Autodesk Fusion 360 part; units mm, degrees
(part 2 of 3)
  arc A16 (-17.9906, -30.6144) -> (-8.9264, -34.3689) centre (0, 0) ccw
  arc A17 (-7.7732, -36.2381) -> (-8.9264, -34.3689) centre (-9.3255, -35.9054) ccw
  line L8 (-7.7732, -36.2381) -> (-10.0097, -46.6751)
  spline S8 degree 5 poles (-10.0097, -46.6751) (-10.0198, -46.7226) (-10.0383, -46.8178) (-10.0605, -46.9612) (-10.0796, -47.1537) (-10.0893, -47.3962) (-10.0891, -47.6398) (-10.0829, -47.8842) (-10.0736, -48.129) (-10.0619, -48.374) (-10.0476, -48.6191) (-10.0296, -48.8645) (-10.007, -49.1102) (-9.9792, -49.3562) (-9.9463, -49.6025) (-9.9089, -49.849) (-9.8676, -50.0955) (-9.8231, -50.3422) (-9.7758, -50.5887) (-9.7255, -50.8353) (-9.6724, -51.0817) (-9.6161, -51.3281) (-9.5567, -51.5744) (-9.4939, -51.8206) (-9.428, -52.0667) (-9.3591, -52.3127) (-9.2873, -52.5584) (-9.2128, -52.804) (-9.1355, -53.0494) (-9.0557, -53.2944) (-8.9732, -53.5393) (-8.8881, -53.7839) (-8.8003, -54.0281) (-8.71, -54.2721) (-8.617, -54.5158) (-8.5215, -54.7591) (-8.4236, -55.0021) (-8.3232, -55.2447) (-8.2204, -55.487) (-8.1152, -55.7288) (-8.0077, -55.9702) (-7.8978, -56.2112) (-7.7856, -56.4518) (-7.6711, -56.6919) (-7.5543, -56.9315) (-7.4353, -57.1707) (-7.314, -57.4094) (-7.1905, -57.6476) (-7.0648, -57.8853) (-6.937, -58.1224) (-6.807, -58.3591) (-6.6749, -58.5951) (-6.5406, -58.8307) (-6.4043, -59.0656) (-6.2659, -59.3) (-6.1254, -59.5337) (-5.9828, -59.7669) (-5.8383, -59.9994) (-5.6917, -60.2314) (-5.5431, -60.4627) (-5.3925, -60.6933) (-5.24, -60.9233) (-5.0855, -61.1526) (-4.929, -61.3813) (-4.7706, -61.6093) (-4.6103, -61.8365) (-4.4481, -62.0631) (-4.2841, -62.2889) (-4.1181, -62.5141) (-3.9503, -62.7384) (-3.7806, -62.9621) (-3.6434, -63.1404) (-3.5397, -63.2738) (-3.4702, -63.3626) (-3.4353, -63.407) knots 0 0 0 0 0 0 0.01428571 0.02857143 0.04285714 0.05714286 0.07142857 0.08571429 0.1 0.11428571 0.12857143 0.14285714 0.15714286 0.17142857 0.18571429 0.2 0.21428571 0.22857143 0.24285714 0.25714286 0.27142857 0.28571429 0.3 0.31428571 0.32857143 0.34285714 0.35714286 0.37142857 0.38571429 0.4 0.41428571 0.42857143 0.44285714 0.45714286 0.47142857 0.48571429 0.5 0.51428571 0.52857143 0.54285714 0.55714286 0.57142857 0.58571429 0.6 0.61428571 0.62857143 0.64285714 0.65714286 0.67142857 0.68571429 0.7 0.71428571 0.72857143 0.74285714 0.75714286 0.77142857 0.78571429 0.8 0.81428571 0.82857143 0.84285714 0.85714286 0.87142857 0.88571429 0.9 0.91428571 0.92857143 0.94285714 0.95714286 0.97142857 0.98571429 1 1 1 1 1 1
  arc A18 (-3.4353, -63.407) -> (3.4353, -63.407) centre (0, 0) ccw
  spline S9 degree 5 poles (10.0097, -46.6751) (10.0198, -46.7226) (10.0383, -46.8178) (10.0605, -46.9612) (10.0796, -47.1537) (10.0893, -47.3962) (10.0891, -47.6398) (10.0829, -47.8842) (10.0736, -48.129) (10.0619, -48.374) (10.0476, -48.6191) (10.0296, -48.8645) (10.007, -49.1102) (9.9792, -49.3562) (9.9463, -49.6025) (9.9089, -49.849) (9.8676, -50.0955) (9.8231, -50.3422) (9.7758, -50.5887) (9.7255, -50.8353) (9.6724, -51.0817) (9.6161, -51.3281) (9.5567, -51.5744) (9.4939, -51.8206) (9.428, -52.0667) (9.3591, -52.3127) (9.2873, -52.5584) (9.2128, -52.804) (9.1355, -53.0494) (9.0557, -53.2944) (8.9732, -53.5393) (8.8881, -53.7839) (8.8003, -54.0281) (8.71, -54.2721) (8.617, -54.5158) (8.5215, -54.7591) (8.4236, -55.0021) (8.3232, -55.2447) (8.2204, -55.487) (8.1152, -55.7288) (8.0077, -55.9702) (7.8978, -56.2112) (7.7856, -56.4518) (7.6711, -56.6919) (7.5543, -56.9315) (7.4353, -57.1707) (7.314, -57.4094) (7.1905, -57.6476) (7.0648, -57.8853) (6.937, -58.1224) (6.807, -58.3591) (6.6749, -58.5951) (6.5406, -58.8307) (6.4043, -59.0656) (6.2659, -59.3) (6.1254, -59.5337) (5.9828, -59.7669) (5.8383, -59.9994) (5.6917, -60.2314) (5.5431, -60.4627) (5.3925, -60.6933) (5.24, -60.9233) (5.0855, -61.1526) (4.929, -61.3813) (4.7706, -61.6093) (4.6103, -61.8365) (4.4481, -62.0631) (4.2841, -62.2889) (4.1181, -62.5141) (3.9503, -62.7384) (3.7806, -62.9621) (3.6434, -63.1404) (3.5397, -63.2738) (3.4702, -63.3626) (3.4353, -63.407) knots 0 0 0 0 0 0 0.01428571 0.02857143 0.04285714 0.05714286 0.07142857 0.08571429 0.1 0.11428571 0.12857143 0.14285714 0.15714286 0.17142857 0.18571429 0.2 0.21428571 0.22857143 0.24285714 0.25714286 0.27142857 0.28571429 0.3 0.31428571 0.32857143 0.34285714 0.35714286 0.37142857 0.38571429 0.4 0.41428571 0.42857143 0.44285714 0.45714286 0.47142857 0.48571429 0.5 0.51428571 0.52857143 0.54285714 0.55714286 0.57142857 0.58571429 0.6 0.61428571 0.62857143 0.64285714 0.65714286 0.67142857 0.68571429 0.7 0.71428571 0.72857143 0.74285714 0.75714286 0.77142857 0.78571429 0.8 0.81428571 0.82857143 0.84285714 0.85714286 0.87142857 0.88571429 0.9 0.91428571 0.92857143 0.94285714 0.95714286 0.97142857 0.98571429 1 1 1 1 1 1
  line L9 (10.0097, -46.6751) -> (7.7732, -36.2381)
  arc A19 (8.9264, -34.3689) -> (7.7732, -36.2381) centre (9.3255, -35.9054) ccw
  arc A20 (8.9264, -34.3689) -> (17.9906, -30.6144) centre (0, 0) ccw
  arc A21 (20.1277, -31.1207) -> (17.9906, -30.6144) centre (18.7949, -31.9831) ccw
  line L10 (20.1277, -31.1207) -> (25.9264, -40.0822)
  spline S10 degree 5 poles (25.9264, -40.0822) (25.9528, -40.123) (26.007, -40.2033) (26.0927, -40.3204) (26.2154, -40.4701) (26.3799, -40.6484) (26.5524, -40.8205) (26.7296, -40.989) (26.9092, -41.1554) (27.0907, -41.3204) (27.2742, -41.4836) (27.4604, -41.6444) (27.6501, -41.8022) (27.8437, -41.9565) (28.0411, -42.1074) (28.2419, -42.2552) (28.4454, -42.4004) (28.6513, -42.5433) (28.8591, -42.6841) (29.069, -42.823) (29.2808, -42.9596) (29.4948, -43.0941) (29.711, -43.2262) (29.9295, -43.3559) (30.1501, -43.4833) (30.3728, -43.6085) (30.5973, -43.7315) (30.8237, -43.8525) (31.0517, -43.9714) (31.2815, -44.0882) (31.513, -44.203) (31.7461, -44.3158) (31.9809, -44.4264) (32.2173, -44.5351) (32.4553, -44.6416) (32.6949, -44.7462) (32.936, -44.8487) (33.1785, -44.9493) (33.4225, -45.0479) (33.6679, -45.1445) (33.9146, -45.2392) (34.1627, -45.3319) (34.4122, -45.4227) (34.6629, -45.5115) (34.915, -45.5984) (35.1683, -45.6833) (35.4228, -45.7664) (35.6786, -45.8475) (35.9355, -45.9267) (36.1936, -46.004) (36.4528, -46.0794) (36.7132, -46.1529) (36.9746, -46.2245) (37.2372, -46.2942) (37.5008, -46.362) (37.7654, -46.428) (38.0311, -46.4921) (38.2977, -46.5543) (38.5654, -46.6146) (38.834, -46.6731) (39.1036, -46.7297) (39.3741, -46.7845) (39.6455, -46.8374) (39.9178, -46.8885) (40.191, -46.9377) (40.465, -46.985) (40.7399, -47.0305) (41.0156, -47.0742) (41.2922, -47.1161) (41.5695, -47.1561) (41.8476, -47.1942) (42.0707, -47.2233) (42.2384, -47.2443) (42.3504, -47.2579) (42.4064, -47.2647) knots 0 0 0 0 0 0 0.01428571 0.02857143 0.04285714 0.05714286 0.07142857 0.08571429 0.1 0.11428571 0.12857143 0.14285714 0.15714286 0.17142857 0.18571429 0.2 0.21428571 0.22857143 0.24285714 0.25714286 0.27142857 0.28571429 0.3 0.31428571 0.32857143 0.34285714 0.35714286 0.37142857 0.38571429 0.4 0.41428571 0.42857143 0.44285714 0.45714286 0.47142857 0.48571429 0.5 0.51428571 0.52857143 0.54285714 0.55714286 0.57142857 0.58571429 0.6 0.61428571 0.62857143 0.64285714 0.65714286 0.67142857 0.68571429 0.7 0.71428571 0.72857143 0.74285714 0.75714286 0.77142857 0.78571429 0.8 0.81428571 0.82857143 0.84285714 0.85714286 0.87142857 0.88571429 0.9 0.91428571 0.92857143 0.94285714 0.95714286 0.97142857 0.98571429 1 1 1 1 1 1
  arc A22 (42.4064, -47.2647) -> (47.2647, -42.4064) centre (0, 0) ccw
  spline S11 degree 5 poles (40.0822, -25.9264) (40.123, -25.9528) (40.2033, -26.007) (40.3204, -26.0927) (40.4701, -26.2154) (40.6484, -26.3799) (40.8205, -26.5524) (40.989, -26.7296) (41.1554, -26.9092) (41.3204, -27.0907) (41.4836, -27.2742) (41.6444, -27.4604) (41.8022, -27.6501) (41.9565, -27.8437) (42.1074, -28.0411) (42.2552, -28.2419) (42.4004, -28.4454) (42.5433, -28.6513) (42.6841, -28.8591) (42.823, -29.069) (42.9596, -29.2808) (43.0941, -29.4948) (43.2262, -29.711) (43.3559, -29.9295) (43.4833, -30.1501) (43.6085, -30.3728) (43.7315, -30.5973) (43.8525, -30.8237) (43.9714, -31.0517) (44.0882, -31.2815) (44.203, -31.513) (44.3158, -31.7461) (44.4264, -31.9809) (44.5351, -32.2173) (44.6416, -32.4553) (44.7462, -32.6949) (44.8487, -32.936) (44.9493, -33.1785) (45.0479, -33.4225) (45.1445, -33.6679) (45.2392, -33.9146) (45.3319, -34.1627) (45.4227, -34.4122) (45.5115, -34.6629) (45.5984, -34.915) (45.6833, -35.1683) (45.7664, -35.4228) (45.8475, -35.6786) (45.9267, -35.9355) (46.004, -36.1936) (46.0794, -36.4528) (46.1529, -36.7132) (46.2245, -36.9746) (46.2942, -37.2372) (46.362, -37.5008) (46.428, -37.7654) (46.4921, -38.0311) (46.5543, -38.2977) (46.6146, -38.5654) (46.6731, -38.834) (46.7297, -39.1036) (46.7845, -39.3741) (46.8374, -39.6455) (46.8885, -39.9178) (46.9377, -40.191) (46.985, -40.465) (47.0305, -40.7399) (47.0742, -41.0156) (47.1161, -41.2922) (47.1561, -41.5695) (47.1942, -41.8476) (47.2233, -42.0707) (47.2443, -42.2384) (47.2579, -42.3504) (47.2647, -42.4064) knots 0 0 0 0 0 0 0.01428571 0.02857143 0.04285714 0.05714286 0.07142857 0.08571429 0.1 0.11428571 0.12857143 0.14285714 0.15714286 0.17142857 0.18571429 0.2 0.21428571 0.22857143 0.24285714 0.25714286 0.27142857 0.28571429 0.3 0.31428571 0.32857143 0.34285714 0.35714286 0.37142857 0.38571429 0.4 0.41428571 0.42857143 0.44285714 0.45714286 0.47142857 0.48571429 0.5 0.51428571 0.52857143 0.54285714 0.55714286 0.57142857 0.58571429 0.6 0.61428571 0.62857143 0.64285714 0.65714286 0.67142857 0.68571429 0.7 0.71428571 0.72857143 0.74285714 0.75714286 0.77142857 0.78571429 0.8 0.81428571 0.82857143 0.84285714 0.85714286 0.87142857 0.88571429 0.9 0.91428571 0.92857143 0.94285714 0.95714286 0.97142857 0.98571429 1 1 1 1 1 1
  line L11 (40.0822, -25.9264) -> (31.1207, -20.1277)
  arc A23 (30.6144, -17.9906) -> (31.1207, -20.1277) centre (31.9831, -18.7949) ccw
  arc A24 (30.6144, -17.9906) -> (34.3689, -8.9264) centre (0, 0) ccw
  arc A25 (36.2381, -7.7732) -> (34.3689, -8.9264) centre (35.9054, -9.3255) ccw
  line L12 (36.2381, -7.7732) -> (46.6751, -10.0097)
  spline S12 degree 5 poles (46.6751, -10.0097) (46.7226, -10.0198) (46.8178, -10.0383) (46.9612, -10.0605) (47.1537, -10.0796) (47.3962, -10.0893) (47.6398, -10.0891) (47.8842, -10.0829) (48.129, -10.0736) (48.374, -10.0619) (48.6191, -10.0476) (48.8645, -10.0296) (49.1102, -10.007) (49.3562, -9.9792) (49.6025, -9.9463) (49.849, -9.9089) (50.0955, -9.8676) (50.3422, -9.8231) (50.5887, -9.7758) (50.8353, -9.7255) (51.0817, -9.6724) (51.3281, -9.6161) (51.5744, -9.5567) (51.8206, -9.4939) (52.0667, -9.428) (52.3127, -9.3591) (52.5584, -9.2873) (52.804, -9.2128) (53.0494, -9.1355) (53.2944, -9.0557) (53.5393, -8.9732) (53.7839, -8.8881) (54.0281, -8.8003) (54.2721, -8.71) (54.5158, -8.617) (54.7591, -8.5215) (55.0021, -8.4236) (55.2447, -8.3232) (55.487, -8.2204) (55.7288, -8.1152) (55.9702, -8.0077) (56.2112, -7.8978) (56.4518, -7.7856) (56.6919, -7.6711) (56.9315, -7.5543) (57.1707, -7.4353) (57.4094, -7.314) (57.6476, -7.1905) (57.8853, -7.0648) (58.1224, -6.937) (58.3591, -6.807) (58.5951, -6.6749) (58.8307, -6.5406) (59.0656, -6.4043) (59.3, -6.2659) (59.5337, -6.1254) (59.7669, -5.9828) (59.9994, -5.8383) (60.2314, -5.6917) (60.4627, -5.5431) (60.6933, -5.3925) (60.9233, -5.24) (61.1526, -5.0855) (61.3813, -4.929) (61.6093, -4.7706) (61.8365, -4.6103) (62.0631, -4.4481) (62.2889, -4.2841) (62.5141, -4.1181) (62.7384, -3.9503) (62.9621, -3.7806) (63.1404, -3.6434) (63.2738, -3.5397) (63.3626, -3.4702) (63.407, -3.4353) knots 0 0 0 0 0 0 0.01428571 0.02857143 0.04285714 0.05714286 0.07142857 0.08571429 0.1 0.11428571 0.12857143 0.14285714 0.15714286 0.17142857 0.18571429 0.2 0.21428571 0.22857143 0.24285714 0.25714286 0.27142857 0.28571429 0.3 0.31428571 0.32857143 0.34285714 0.35714286 0.37142857 0.38571429 0.4 0.41428571 0.42857143 0.44285714 0.45714286 0.47142857 0.48571429 0.5 0.51428571 0.52857143 0.54285714 0.55714286 0.57142857 0.58571429 0.6 0.61428571 0.62857143 0.64285714 0.65714286 0.67142857 0.68571429 0.7 0.71428571 0.72857143 0.74285714 0.75714286 0.77142857 0.78571429 0.8 0.81428571 0.82857143 0.84285714 0.85714286 0.87142857 0.88571429 0.9 0.91428571 0.92857143 0.94285714 0.95714286 0.97142857 0.98571429 1 1 1 1 1 1
  arc A26 (63.407, -3.4353) -> (63.407, 3.4353) centre (0, 0) ccw
  spline S13 degree 5 poles (46.6751, 10.0097) (46.7226, 10.0198) (46.8178, 10.0383) (46.9612, 10.0605) (47.1537, 10.0796) (47.3962, 10.0893) (47.6398, 10.0891) (47.8842, 10.0829) (48.129, 10.0736) (48.374, 10.0619) (48.6191, 10.0476) (48.8645, 10.0296) (49.1102, 10.007) (49.3562, 9.9792) (49.6025, 9.9463) (49.849, 9.9089) (50.0955, 9.8676) (50.3422, 9.8231) (50.5887, 9.7758) (50.8353, 9.7255) (51.0817, 9.6724) (51.3281, 9.6161) (51.5744, 9.5567) (51.8206, 9.4939) (52.0667, 9.428) (52.3127, 9.3591) (52.5584, 9.2873) (52.804, 9.2128) (53.0494, 9.1355) (53.2944, 9.0557) (53.5393, 8.9732) (53.7839, 8.8881) (54.0281, 8.8003) (54.2721, 8.71) (54.5158, 8.617) (54.7591, 8.5215) (55.0021, 8.4236) (55.2447, 8.3232) (55.487, 8.2204) (55.7288, 8.1152) (55.9702, 8.0077) (56.2112, 7.8978) (56.4518, 7.7856) (56.6919, 7.6711) (56.9315, 7.5543) (57.1707, 7.4353) (57.4094, 7.314) (57.6476, 7.1905) (57.8853, 7.0648) (58.1224, 6.937) (58.3591, 6.807) (58.5951, 6.6749) (58.8307, 6.5406) (59.0656, 6.4043) (59.3, 6.2659) (59.5337, 6.1254) (59.7669, 5.9828) (59.9994, 5.8383) (60.2314, 5.6917) (60.4627, 5.5431) (60.6933, 5.3925) (60.9233, 5.24) (61.1526, 5.0855) (61.3813, 4.929) (61.6093, 4.7706) (61.8365, 4.6103) (62.0631, 4.4481) (62.2889, 4.2841) (62.5141, 4.1181) (62.7384, 3.9503) (62.9621, 3.7806) (63.1404, 3.6434) (63.2738, 3.5397) (63.3626, 3.4702) (63.407, 3.4353) knots 0 0 0 0 0 0 0.01428571 0.02857143 0.04285714 0.05714286 0.07142857 0.08571429 0.1 0.11428571 0.12857143 0.14285714 0.15714286 0.17142857 0.18571429 0.2 0.21428571 0.22857143 0.24285714 0.25714286 0.27142857 0.28571429 0.3 0.31428571 0.32857143 0.34285714 0.35714286 0.37142857 0.38571429 0.4 0.41428571 0.42857143 0.44285714 0.45714286 0.47142857 0.48571429 0.5 0.51428571 0.52857143 0.54285714 0.55714286 0.57142857 0.58571429 0.6 0.61428571 0.62857143 0.64285714 0.65714286 0.67142857 0.68571429 0.7 0.71428571 0.72857143 0.74285714 0.75714286 0.77142857 0.78571429 0.8 0.81428571 0.82857143 0.84285714 0.85714286 0.87142857 0.88571429 0.9 0.91428571 0.92857143 0.94285714 0.95714286 0.97142857 0.98571429 1 1 1 1 1 1
  line L13 (46.6751, 10.0097) -> (36.2381, 7.7732)
  arc A27 (34.3689, 8.9264) -> (36.2381, 7.7732) centre (35.9054, 9.3255) ccw
  arc A28 (34.3689, 8.9264) -> (30.6144, 17.9906) centre (0, 0) ccw
  arc A29 (31.1207, 20.1277) -> (30.6144, 17.9906) centre (31.9831, 18.7949) ccw
  line L14 (31.1207, 20.1277) -> (40.0822, 25.9264)
  spline S14 degree 5 poles (40.0822, 25.9264) (40.123, 25.9528) (40.2033, 26.007) (40.3204, 26.0927) (40.4701, 26.2154) (40.6484, 26.3799) (40.8205, 26.5524) (40.989, 26.7296) (41.1554, 26.9092) (41.3204, 27.0907) (41.4836, 27.2742) (41.6444, 27.4604) (41.8022, 27.6501) (41.9565, 27.8437) (42.1074, 28.0411) (42.2552, 28.2419) (42.4004, 28.4454) (42.5433, 28.6513) (42.6841, 28.8591) (42.823, 29.069) (42.9596, 29.2808) (43.0941, 29.4948) (43.2262, 29.711) (43.3559, 29.9295) (43.4833, 30.1501) (43.6085, 30.3728) (43.7315, 30.5973) (43.8525, 30.8237) (43.9714, 31.0517) (44.0882, 31.2815) (44.203, 31.513) (44.3158, 31.7461) (44.4264, 31.9809) (44.5351, 32.2173) (44.6416, 32.4553) (44.7462, 32.6949) (44.8487, 32.936) (44.9493, 33.1785) (45.0479, 33.4225) (45.1445, 33.6679) (45.2392, 33.9146) (45.3319, 34.1627) (45.4227, 34.4122) (45.5115, 34.6629) (45.5984, 34.915) (45.6833, 35.1683) (45.7664, 35.4228) (45.8475, 35.6786) (45.9267, 35.9355) (46.004, 36.1936) (46.0794, 36.4528) (46.1529, 36.7132) (46.2245, 36.9746) (46.2942, 37.2372) (46.362, 37.5008) (46.428, 37.7654) (46.4921, 38.0311) (46.5543, 38.2977) (46.6146, 38.5654) (46.6731, 38.834) (46.7297, 39.1036) (46.7845, 39.3741) (46.8374, 39.6455) (46.8885, 39.9178) (46.9377, 40.191) (46.985, 40.465) (47.0305, 40.7399) (47.0742, 41.0156) (47.1161, 41.2922) (47.1561, 41.5695) (47.1942, 41.8476) (47.2233, 42.0707) (47.2443, 42.2384) (47.2579, 42.3504) (47.2647, 42.4064) knots 0 0 0 0 0 0 0.01428571 0.02857143 0.04285714 0.05714286 0.07142857 0.08571429 0.1 0.11428571 0.12857143 0.14285714 0.15714286 0.17142857 0.18571429 0.2 0.21428571 0.22857143 0.24285714 0.25714286 0.27142857 0.28571429 0.3 0.31428571 0.32857143 0.34285714 0.35714286 0.37142857 0.38571429 0.4 0.41428571 0.42857143 0.44285714 0.45714286 0.47142857 0.48571429 0.5 0.51428571 0.52857143 0.54285714 0.55714286 0.57142857 0.58571429 0.6 0.61428571 0.62857143 0.64285714 0.65714286 0.67142857 0.68571429 0.7 0.71428571 0.72857143 0.74285714 0.75714286 0.77142857 0.78571429 0.8 0.81428571 0.82857143 0.84285714 0.85714286 0.87142857 0.88571429 0.9 0.91428571 0.92857143 0.94285714 0.95714286 0.97142857 0.98571429 1 1 1 1 1 1
  arc A30 (47.2647, 42.4064) -> (42.4064, 47.2647) centre (0, 0) ccw
  spline S15 degree 5 poles (25.9264, 40.0822) (25.9528, 40.123) (26.007, 40.2033) (26.0927, 40.3204) (26.2154, 40.4701) (26.3799, 40.6484) (26.5524, 40.8205) (26.7296, 40.989) (26.9092, 41.1554) (27.0907, 41.3204) (27.2742, 41.4836) (27.4604, 41.6444) (27.6501, 41.8022) (27.8437, 41.9565) (28.0411, 42.1074) (28.2419, 42.2552) (28.4454, 42.4004) (28.6513, 42.5433) (28.8591, 42.6841) (29.069, 42.823) (29.2808, 42.9596) (29.4948, 43.0941) (29.711, 43.2262) (29.9295, 43.3559) (30.1501, 43.4833) (30.3728, 43.6085) (30.5973, 43.7315) (30.8237, 43.8525) (31.0517, 43.9714) (31.2815, 44.0882) (31.513, 44.203) (31.7461, 44.3158) (31.9809, 44.4264) (32.2173, 44.5351) (32.4553, 44.6416) (32.6949, 44.7462) (32.936, 44.8487) (33.1785, 44.9493) (33.4225, 45.0479) (33.6679, 45.1445) (33.9146, 45.2392) (34.1627, 45.3319) (34.4122, 45.4227) (34.6629, 45.5115) (34.915, 45.5984) (35.1683, 45.6833) (35.4228, 45.7664) (35.6786, 45.8475) (35.9355, 45.9267) (36.1936, 46.004) (36.4528, 46.0794) (36.7132, 46.1529) (36.9746, 46.2245) (37.2372, 46.2942) (37.5008, 46.362) (37.7654, 46.428) (38.0311, 46.4921) (38.2977, 46.5543) (38.5654, 46.6146) (38.834, 46.6731) (39.1036, 46.7297) (39.3741, 46.7845) (39.6455, 46.8374) (39.9178, 46.8885) (40.191, 46.9377) (40.465, 46.985) (40.7399, 47.0305) (41.0156, 47.0742) (41.2922, 47.1161) (41.5695, 47.1561) (41.8476, 47.1942) (42.0707, 47.2233) (42.2384, 47.2443) (42.3504, 47.2579) (42.4064, 47.2647) knots 0 0 0 0 0 0 0.01428571 0.02857143 0.04285714 0.05714286 0.07142857 0.08571429 0.1 0.11428571 0.12857143 0.14285714 0.15714286 0.17142857 0.18571429 0.2 0.21428571 0.22857143 0.24285714 0.25714286 0.27142857 0.28571429 0.3 0.31428571 0.32857143 0.34285714 0.35714286 0.37142857 0.38571429 0.4 0.41428571 0.42857143 0.44285714 0.45714286 0.47142857 0.48571429 0.5 0.51428571 0.52857143 0.54285714 0.55714286 0.57142857 0.58571429 0.6 0.61428571 0.62857143 0.64285714 0.65714286 0.67142857 0.68571429 0.7 0.71428571 0.72857143 0.74285714 0.75714286 0.77142857 0.78571429 0.8 0.81428571 0.82857143 0.84285714 0.85714286 0.87142857 0.88571429 0.9 0.91428571 0.92857143 0.94285714 0.95714286 0.97142857 0.98571429 1 1 1 1 1 1
  line L15 (25.9264, 40.0822) -> (20.1277, 31.1207)
  arc A31 (17.9906, 30.6144) -> (20.1277, 31.1207) centre (18.7949, 31.9831) ccw
  arc A32 (17.9906, 30.6144) -> (8.9264, 34.3689) centre (0, 0) ccw
  circle A33 centre (0, 0) radius 7
  circle A34 centre (0, 0) radius 10
  line L16 (0, 13) -> (0, -12)
  circle A35 centre (0, 0) radius 27.5
  circle A36 centre (0, 0) radius 15
  line L17 (0, 0) -> (-5.1303, 14.0954)
  line L18 (0, 0) -> (5.1303, 14.0954)
  line L19 (-5.1303, 14.0954) -> (-9.4056, 25.8415)
  line L20 (5.1303, 14.0954) -> (9.4056, 25.8415)
  line L21 (-14.7721, 2.6047) -> (-27.0822, 4.7753)
  line L22 (-9.6418, 11.4907) -> (-17.6767, 21.0662)
  line L23 (-9.6418, -11.4907) -> (-17.6767, -21.0662)
  line L24 (-14.7721, -2.6047) -> (-27.0822, -4.7753)
  line L25 (5.1303, -14.0954) -> (9.4056, -25.8415)
  line L26 (-5.1303, -14.0954) -> (-9.4056, -25.8415)
  line L27 (14.7721, -2.6047) -> (27.0822, -4.7753)
  line L28 (9.6418, -11.4907) -> (17.6767, -21.0662)
  line L29 (9.6418, 11.4907) -> (17.6767, 21.0662)
  line L30 (14.7721, 2.6047) -> (27.0822, 4.7753)
  point P0 (0, 7)
  dimension "d25" = 14
  dimension "d30" = 3
  dimension "d37" = 55
  dimension "d38" = 30
  dimension "d39" = 40
  dimension "d40" = 20
  dimension "d42" = 360
  constraint concentric A0 A33
  constraint vertical L16
  constraint coincident A0.centre L16
  constraint coincident L16 P0
  constraint coincident A33 P0
  constraint concentric A33 A35
  constraint concentric A33 A36
  constraint coincident A0.centre A2.centre
  constraint coincident A35 L19.end
  constraint coincident A35 L20.end
  constraint coincident A36 L17.end
  constraint coincident A36 L18.end
  measures "d25" diameter of A33
  measures "d37" diameter of A35
  measures "d38" diameter of A36
  measures "d39" angle of L17 L18
  measures "d40" angle of L16 L18
extrude "Extrude3" cut sketch "Sketch1 (3)" against normal up to surface (32.7 mm away) contours A0 A33 L16 L18 | A0 A33 L16 L18 | A0 A33 L16 L17 | A0 A33 L16 L17 bodies 1 in component "Spur Gear (8 teeth)"
extrude "Extrude3'" cut sketch "Sketch1 (3)" against normal up to surface (32.7 mm away) contours A0 A33 L16 L18 | A0 A33 L16 L18 | A0 A33 L16 L17 | A0 A33 L16 L17 bodies 2 in component "Spur Gear (4 teeth)"
extrude "Extrude4" add sketch "Sketch1 (3)" against normal up to surface (32.7 mm away) contours A33 A34 L16 L18 | A33 A34 L16 L18 | A33 A34 L16 L17 | A33 A34 L16 L17 bodies 1 in component "Spur Gear (8 teeth)"
extrude "Extrude6" cut sketch "Sketch1 (3)" against normal up to surface (12.7 mm away) contours A35 A36 L19 L20 | A35 A36 L29 L30 | A35 A36 L21 L22 | A35 A36 L27 L28 | A35 A36 L23 L24 | A35 A36 L25 L26 bodies 1 in component "Spur Gear (8 teeth)"
component "Spur Gear (8 teeth)" placed x (1, 0, 0) y (0, 1, 0) z (0, 0, 1) at (0, 0, 0)
component "Spur Gear (4 teeth)" placed x (1, 0, 0) y (0, 1, 0) z (0, 0, 1) at (0, 0, 0)

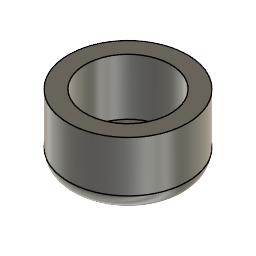
design "Cap 2"
Autodesk Fusion 360 part; units mm, degrees
sketch "Sketch1" plane through (0, 0, 0) normal (0, 0, 1) x (1, 0, 0)
  circle A0 centre (0, 0) radius 7.55
  circle A1 centre (0, 0) radius 10.55
  dimension "d1" = 3
  dimension "d2" = 15.1
  constraint coincident A0.centre A1.centre
  measures "d2" diameter of A0
extrude "Extrude1" add sketch "Sketch1" along normal blind 10
extrude "Extrude2" add sketch "Sketch1" against normal blind 2 contours A0 | A1
fillet "Fillet1" radius 3 1 edges at (-9.8361, 3.815, -2)

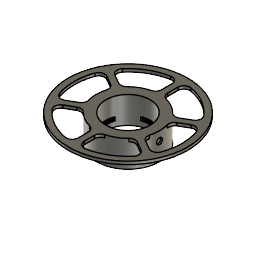
design "Font Reel"
part number: 2026-01-12-12-34-36-869
Autodesk Fusion 360 part; units mm, degrees
sketch "Sketch1" plane through (0, 0, 0) normal (0, 0, 1) x (1, 0, 0)
  circle A0 centre (0, 0) radius 90
  circle A1 centre (0, 0) radius 50
  circle A2 centre (0, 0) radius 53
  circle A3 centre (0, 0) radius 100
  line L0 (-5, 89.861) -> (-5, 52.7636)
  line L1 (5, 89.861) -> (5, 52.7636)
  line L2 (0, 110) -> (0, -110)
  line L3 (-80.3219, 40.6004) -> (-48.1946, 22.0517)
  line L4 (-75.3219, 49.2606) -> (-43.1946, 30.7119)
  line L5 (-75.3219, -49.2606) -> (-43.1946, -30.7119)
  line L6 (-80.3219, -40.6004) -> (-48.1946, -22.0517)
  line L7 (5, -89.861) -> (5, -52.7636)
  line L8 (-5, -89.861) -> (-5, -52.7636)
  line L9 (80.3219, -40.6004) -> (48.1946, -22.0517)
  line L10 (75.3219, -49.2606) -> (43.1946, -30.7119)
  line L11 (75.3219, 49.2606) -> (43.1946, 30.7119)
  line L12 (80.3219, 40.6004) -> (48.1946, 22.0517)
  circle A4 centre (0, 0) radius 40
  line L13 (-1.5, 49.9775) -> (-1.5, 39.9719)
  line L14 (1.5, 49.9775) -> (1.5, 39.9719)
  line L15 (-42.5318, 26.2878) -> (-33.8667, 21.285)
  line L16 (-44.0318, 23.6897) -> (-35.3667, 18.6869)
  line L17 (-44.0318, -23.6897) -> (-35.3667, -18.6869)
  line L18 (-42.5318, -26.2878) -> (-33.8667, -21.285)
  line L19 (-1.5, -49.9775) -> (-1.5, -39.9719)
  line L20 (1.5, -49.9775) -> (1.5, -39.9719)
  line L21 (42.5318, -26.2878) -> (33.8667, -21.285)
  line L22 (44.0318, -23.6897) -> (35.3667, -18.6869)
  line L23 (44.0318, 23.6897) -> (35.3667, 18.6869)
  line L24 (42.5318, 26.2878) -> (33.8667, 21.285)
  circle A5 centre (0, 0) radius 47
  circle A6 centre (0, 0) radius 37
  circle A7 centre (0, 0) radius 35.5
  line L25 (12.1417, 33.3591) -> (0, 0)
  line L26 (-12.1417, 33.3591) -> (0, 0)
  line L27 (12.1417, 33.3591) -> (12.6547, 34.7686)
  line L28 (-12.1417, 33.3591) -> (-12.6547, 34.7686)
  line L29 (-33.3591, 12.1417) -> (-34.7686, 12.6547)
  line L30 (-33.3591, -12.1417) -> (-34.7686, -12.6547)
  line L31 (-12.1417, -33.3591) -> (-12.6547, -34.7686)
  line L32 (12.1417, -33.3591) -> (12.6547, -34.7686)
  line L33 (33.3591, -12.1417) -> (34.7686, -12.6547)
  line L34 (33.3591, 12.1417) -> (34.7686, 12.6547)
  line L35 (-10.1986, 35.5667) -> (-9.7851, 34.1248)
  line L36 (-9.7851, 34.1248) -> (0, 0)
  line L37 (-35.5667, -10.1986) -> (-34.1248, -9.7851)
  line L38 (10.1986, -35.5667) -> (9.7851, -34.1248)
  line L39 (35.5667, 10.1986) -> (34.1248, 9.7851)
  dimension "d1" = 180
  dimension "d2" = 100
  dimension "d3" = 3
  dimension "d8" = 10
  dimension "d9" = 10
  dimension "d11" = 360
  dimension "d18" = -10
  dimension "d19" = 3
  dimension "d21" = 360
  dimension "d24" = -3
  dimension "d28" = -3
  dimension "d44" = -1.5
  dimension "d47" = 40
  dimension "d48" = 20
  dimension "d50" = 360
  dimension "d54" = 4
  dimension "d56" = 360
  constraint coincident A0.centre A1.centre
  constraint concentric A0 A1
  constraint coincident A0 L0.start
  constraint coincident A2 L0.end
  constraint vertical L0
  constraint coincident A0 L1.start
  constraint coincident A2 L1.end
  constraint parallel L0 L1
  constraint vertical L2
  constraint symmetric L0 L1 L2
  constraint coincident L2 A0.centre
  constraint coincident A1 L13.start
  constraint coincident A4 L13.end
  constraint parallel L2 L13
  constraint coincident A1 L14.start
  constraint coincident A4 L14.end
  constraint parallel L2 L14
  constraint symmetric L2 L13 L14
  constraint coincident A7 L25.start
  constraint coincident A7 L26.start
  constraint coincident A6 L27.end
  constraint parallel L25 L27
  constraint coincident A6 L28.end
  constraint parallel L26 L28
  constraint coincident A6 L35.start
  constraint coincident A7 L35.end
  measures "d1" diameter of A0
  measures "d2" diameter of A1
  measures "d9" distance of L0 L1
  measures "d19" distance of L13 L14
  measures "d47" angle of L25 L26
  measures "d48" angle of L2 L26
  measures "d54" angle of L26 L35
extrude "Extrude3" add sketch "Sketch1" along normal blind 5 contours A0 A3 L2 | A0 A2 L11 L12 | A0 A2 L9 L10 | A1 A2 L2 | A0 A2 L1 L2 | A0 A2 L2 L7 | A0 A2 L0 L2 | A0 A3 L2 | A0 A2 L2 L8 | A1 A2 L2 | A0 A2 L3 L4 | A1 L2 L13 A5 | A1 L2 L14 A5 | A0 A2 L5 L6 | A1 L2 L20 A5 | A1 L2 L19 A5 | A1 L14 L24 A5 | A1 L13 L15 A5 | L2 A4 L14 A5 | L2 A4 L13 A5 | A1 L18 L19 A5 | A1 L20 L21 A5 | L2 A4 L19 A5 | L2 A4 L20 A5 | A1 L23 L24 A5 | A4 L14 L24 A5 | A1 L15 L16 A5 | A4 L13 L15 A5 | L2 A4 A6 | L2 A4 A6 | A1 L17 L18 A5 | A4 L18 L19 A5 | A1 L21 L22 A5 | A4 L20 L21 A5 | A1 L22 L23 A5 | A4 L23 L24 A5 | A1 L16 L17 A5 | A4 L15 L16 A5 | A4 L17 L18 A5 | A4 L21 L22 A5 | A4 L22 L23 A5 | A4 L16 L17 A5
extrude "Extrude9" add sketch "Sketch1" against normal blind 40 contours A1 A2 L2 | A1 A2 L2 | A1 L2 L13 A5 | A1 L2 L14 A5 | A1 L2 L20 A5 | A1 L2 L19 A5 | L2 A4 L14 A5 | L2 A4 L13 A5 | L2 A4 L19 A5 | L2 A4 L20 A5 | A1 L23 L24 A5 | A1 L15 L16 A5 | L2 A4 A6 | L2 A4 A6 | A1 L17 L18 A5 | A1 L21 L22 A5 | A4 L23 L24 A5 | A4 L15 L16 A5 | A4 L17 L18 A5 | A4 L21 L22 A5
extrude "Extrude10" cut sketch "Sketch1" along normal blind 5 from surface at -40 contours A1 L2 L13 A5 | A1 L2 L14 A5 | A1 L2 L20 A5 | A1 L2 L19 A5 | A1 L23 L24 A5 | A1 L15 L16 A5 | A1 L17 L18 A5 | A1 L21 L22 A5
fillet "Fillet2" radius 10 24 edges at (43.1946, 30.7119, 2.5) (48.1946, 22.0517, 2.5) (48.1946, -22.0517, 2.5) (43.1946, -30.7119, 2.5) (5, -52.7636, 2.5) (-5, -52.7636, 2.5) (-43.1946, -30.7119, 2.5) (-48.1946, -22.0517, 2.5) (-48.1946, 22.0517, 2.5) (-43.1946, 30.7119, 2.5) (-5, 52.7636, 2.5) (5, 52.7636, 2.5) (75.3219, 49.2606, 2.5) (-5, 89.861, 2.5) (5, 89.861, 2.5) (-75.3219, 49.2606, 2.5) (-80.3219, 40.6004, 2.5) (-80.3219, -40.6004, 2.5) (-75.3219, -49.2606, 2.5) (-5, -89.861, 2.5) (5, -89.861, 2.5) (75.3219, -49.2606, 2.5) (80.3219, -40.6004, 2.5) (80.3219, 40.6004, 2.5)
extrude "Extrude11" add sketch "Sketch1" along normal blind 5 from surface at -29.8 contours L2 A6 A7 L27 | L2 A6 A7 L35 | L2 A6 A7 L31 | L2 A6 A7 L38 | A6 A7 L28 L35 | A6 A7 L32 L38 | A6 A7 L34 L39 | A6 A7 L30 L37 | A6 A7 L33 L39 | A6 A7 L29 L37
extrude "Extrude12" cut sketch "Sketch1" along normal blind 2 from surface at -28.3 contours L2 A6 A7 L27 | L2 A6 A7 L35 | L2 A6 A7 L31 | L2 A6 A7 L38 | A6 A7 L33 L39 | A6 A7 L29 L37
fillet "Fillet4" radius 2 6 edges at (40.7032, -23.5, -40) (40.7032, 23.5, -40) (0, 47, -40) (-40.7032, 23.5, -40) (-40.7032, -23.5, -40) (0, -47, -40)
sketch "Sketch3" plane through (0, 0, 0) normal (1, 0, 0) x (0, 1, 0)
  circle A0 centre (0, -10) radius 5
  line L0 (0, 0) -> (0, -10)
  dimension "d67" = 10
  dimension "d68" = 10
  constraint coincident L0.start origin
  constraint coincident A0.centre L0.end
  constraint vertical L0
  measures "d67" diameter of A0
  measures "d68" distance of L0.start A0.centre
extrude "Extrude15" cut sketch "Sketch3" along normal through all

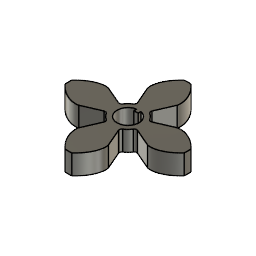
design "Gear 3"
description: Spur Gear; Module: 12.700000; Num Teeth: 4; Pressure Angle: 20.000000; Backlash: 0.00 mm
Autodesk Fusion 360 part; units mm, degrees
sketch "Sketch1" plane through (0, 0, 0) normal (0, 0, 1) x (1, 0, 0) in component "Spur Gear (4 teeth)"
  circle A0 centre (0, 0) radius 10.1092
  circle A1 centre (0, 0) radius 6.35
extrude "Extrude1" add sketch "Sketch1" along normal blind 12.7 in component "Spur Gear (4 teeth)"
sketch "Sketch2" plane through (0, 0, 0) normal (0, 0, 1) x (1, 0, 0) in component "Spur Gear (4 teeth)"
  spline S0 degree 5 poles (21.9128, -9.4616) (21.9552, -9.4799) (22.0407, -9.5141) (22.1712, -9.5583) (22.3491, -9.6037) (22.5768, -9.6426) (22.8081, -9.6692) (23.0414, -9.6889) (23.2758, -9.7048) (23.5109, -9.7174) (23.7467, -9.7262) (23.9837, -9.7295) (24.2219, -9.7262) (24.4615, -9.7158) (24.7023, -9.6987) (24.9439, -9.6758) (25.1862, -9.648) (25.4288, -9.6159) (25.6717, -9.5798) (25.9149, -9.5397) (26.1582, -9.4952) (26.4018, -9.4462) (26.6456, -9.3926) (26.8896, -9.3344) (27.1337, -9.2719) (27.3777, -9.2051) (27.6217, -9.1343) (27.8655, -9.0596) (28.109, -8.9811) (28.3523, -8.8987) (28.5954, -8.8125) (28.838, -8.7225) (29.0803, -8.6286) (29.3222, -8.531) (29.5637, -8.4296) (29.8046, -8.3246) (30.045, -8.216) (30.2848, -8.1038) (30.5239, -7.9882) (30.7623, -7.869) (31.0001, -7.7465) (31.2371, -7.6205) (31.4733, -7.491) (31.7087, -7.3583) (31.9432, -7.2221) (32.1769, -7.0827) (32.4096, -6.9401) (32.6414, -6.7942) (32.8722, -6.6451) (33.1019, -6.4928) (33.3306, -6.3374) (33.5583, -6.1789) (33.7848, -6.0173) (34.0102, -5.8526) (34.2343, -5.6849) (34.4573, -5.5142) (34.6791, -5.3405) (34.8996, -5.1639) (35.1188, -4.9843) (35.3367, -4.8018) (35.5532, -4.6165) (35.7684, -4.4283) (35.9823, -4.2373) (36.1947, -4.0436) (36.4056, -3.847) (36.6151, -3.6477) (36.823, -3.4457) (37.0294, -3.241) (37.2343, -3.0337) (37.4376, -2.8237) (37.6393, -2.6111) (37.7995, -2.4389) (37.9189, -2.3086) (37.9982, -2.2212) (38.0377, -2.1774) knots 0 0 0 0 0 0 0.01428571 0.02857143 0.04285714 0.05714286 0.07142857 0.08571429 0.1 0.11428571 0.12857143 0.14285714 0.15714286 0.17142857 0.18571429 0.2 0.21428571 0.22857143 0.24285714 0.25714286 0.27142857 0.28571429 0.3 0.31428571 0.32857143 0.34285714 0.35714286 0.37142857 0.38571429 0.4 0.41428571 0.42857143 0.44285714 0.45714286 0.47142857 0.48571429 0.5 0.51428571 0.52857143 0.54285714 0.55714286 0.57142857 0.58571429 0.6 0.61428571 0.62857143 0.64285714 0.65714286 0.67142857 0.68571429 0.7 0.71428571 0.72857143 0.74285714 0.75714286 0.77142857 0.78571429 0.8 0.81428571 0.82857143 0.84285714 0.85714286 0.87142857 0.88571429 0.9 0.91428571 0.92857143 0.94285714 0.95714286 0.97142857 0.98571429 1 1 1 1 1 1
  spline S1 degree 5 poles (21.9128, 9.4616) (21.9552, 9.4799) (22.0407, 9.5141) (22.1712, 9.5583) (22.3491, 9.6037) (22.5768, 9.6426) (22.8081, 9.6692) (23.0414, 9.6889) (23.2758, 9.7048) (23.5109, 9.7174) (23.7467, 9.7262) (23.9837, 9.7295) (24.2219, 9.7262) (24.4615, 9.7158) (24.7023, 9.6987) (24.9439, 9.6758) (25.1862, 9.648) (25.4288, 9.6159) (25.6717, 9.5798) (25.9149, 9.5397) (26.1582, 9.4952) (26.4018, 9.4462) (26.6456, 9.3926) (26.8896, 9.3344) (27.1337, 9.2719) (27.3777, 9.2051) (27.6217, 9.1343) (27.8655, 9.0596) (28.109, 8.9811) (28.3523, 8.8987) (28.5954, 8.8125) (28.838, 8.7225) (29.0803, 8.6286) (29.3222, 8.531) (29.5637, 8.4296) (29.8046, 8.3246) (30.045, 8.216) (30.2848, 8.1038) (30.5239, 7.9882) (30.7623, 7.869) (31.0001, 7.7465) (31.2371, 7.6205) (31.4733, 7.491) (31.7087, 7.3583) (31.9432, 7.2221) (32.1769, 7.0827) (32.4096, 6.9401) (32.6414, 6.7942) (32.8722, 6.6451) (33.1019, 6.4928) (33.3306, 6.3374) (33.5583, 6.1789) (33.7848, 6.0173) (34.0102, 5.8526) (34.2343, 5.6849) (34.4573, 5.5142) (34.6791, 5.3405) (34.8996, 5.1639) (35.1188, 4.9843) (35.3367, 4.8018) (35.5532, 4.6165) (35.7684, 4.4283) (35.9823, 4.2373) (36.1947, 4.0436) (36.4056, 3.847) (36.6151, 3.6477) (36.823, 3.4457) (37.0294, 3.241) (37.2343, 3.0337) (37.4376, 2.8237) (37.6393, 2.6111) (37.7995, 2.4389) (37.9189, 2.3086) (37.9982, 2.2212) (38.0377, 2.1774) knots 0 0 0 0 0 0 0.01428571 0.02857143 0.04285714 0.05714286 0.07142857 0.08571429 0.1 0.11428571 0.12857143 0.14285714 0.15714286 0.17142857 0.18571429 0.2 0.21428571 0.22857143 0.24285714 0.25714286 0.27142857 0.28571429 0.3 0.31428571 0.32857143 0.34285714 0.35714286 0.37142857 0.38571429 0.4 0.41428571 0.42857143 0.44285714 0.45714286 0.47142857 0.48571429 0.5 0.51428571 0.52857143 0.54285714 0.55714286 0.57142857 0.58571429 0.6 0.61428571 0.62857143 0.64285714 0.65714286 0.67142857 0.68571429 0.7 0.71428571 0.72857143 0.74285714 0.75714286 0.77142857 0.78571429 0.8 0.81428571 0.82857143 0.84285714 0.85714286 0.87142857 0.88571429 0.9 0.91428571 0.92857143 0.94285714 0.95714286 0.97142857 0.98571429 1 1 1 1 1 1
  arc A0 (38.0377, -2.1774) -> (38.0377, 2.1774) centre (0, 0) ccw
  line L0 (9.2718, -4.0074) -> (21.9128, -9.4616)
  line L1 (9.2718, 4.0074) -> (21.9128, 9.4616)
  line L2 (9.2718, -4.0074) -> (9.2718, 4.0074)
  point P0 (22.9255, -9.6784)
  point P1 (24.0052, -9.7278)
  point P2 (25.1271, -9.6541)
  point P3 (26.2802, -9.4701)
  point P4 (27.4564, -9.1817)
  point P5 (28.6488, -8.792)
  point P6 (29.8509, -8.303)
  point P7 (31.0565, -7.7159)
  point P8 (32.2598, -7.0314)
  point P9 (33.4549, -6.2504)
  point P10 (34.636, -5.3736)
  point P11 (35.7973, -4.4018)
  point P12 (36.9331, -3.336)
  point P13 (22.9255, 9.6784)
  point P14 (24.0052, 9.7278)
  point P15 (25.1271, 9.6541)
  point P16 (26.2802, 9.4701)
  point P17 (27.4564, 9.1817)
  point P18 (28.6488, 8.792)
  point P19 (29.8509, 8.303)
  point P20 (31.0565, 7.7159)
  point P21 (32.2598, 7.0314)
  point P22 (33.4549, 6.2504)
  point P23 (34.636, 5.3736)
  point P24 (35.7973, 4.4018)
  point P25 (36.9331, 3.336)
extrude "Extrude2" add sketch "Sketch2" along normal blind 12.7 in component "Spur Gear (4 teeth)"
fillet "Fillet1" radius 1.5875 2 edges at (9.2795, -4.0107, 6.35) (9.2795, 4.0107, 6.35) in component "Spur Gear (4 teeth)"
pattern_circular "C-Pattern1" count 4 over 360 about axis through (0, 0, 0) along (0, 0, 1) of "Extrude2", "Fillet1" in component "Spur Gear (4 teeth)"
sketch "Sketch3" plane through (0, 0, 0) normal (0, 0, 1) x (1, 0, 0) in component "Spur Gear (4 teeth)"
  circle A0 centre (0, 0) radius 25.4 construction